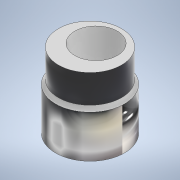
# Autodesk Inventor part: interior
Saved by Autodesk Inventor 2021 (Build 250183000, 183)
## iProperties
Created: 2022-10-29
Part Number: interior
Material: Genérico
Document SubType Name: Modeling
Designer: sergi
Density: 1 g/cm^3
Appearance: Valor por defecto
Author: sergi
Autodesk Inventor part; units mm, degrees
ref_plane "YZ Plane" through (0, 0, 0) normal (1, 0, 0) x (0, 1, 0)
ref_plane "XZ Plane" through (0, 0, 0) normal (0, 1, 0) x (-1, 0, 0)
ref_plane "XY Plane" through (0, 0, 0) normal (0, 0, 1) x (1, 0, 0)
sketch "Boceto1" plane through (0, 0, 0) normal (0, 1, 0) x (-1, 0, 0)
  circle A0 centre (0, 0) radius 4.05
  dimension "d0" = 8.1
  constraints: 1 centre point, 1 coincident
  measures "d0" diameter of A0
extrude "Extrusión1" add sketch "Boceto1" along normal blind 5
sketch "Boceto2" plane through (0, 5, 0) normal (0, 1, 0) x (1, 0, 0)
  circle A0 centre (0, 0) radius 3.715
  dimension "d3" = 7.43
  constraints: 1 centre point, 1 coincident
  measures "d3" diameter of A0
extrude "Extrusión2" add sketch "Boceto2" along normal blind 3.8
fillet "Empalme2" radius 0.5 1 edges at (-3.715, 5, 0)
sketch "Boceto14" plane through (0, 8.8, 0) normal (0, 1, 0) x (1, 0, 0)
  circle A0 centre (0, 0) radius 3.715 projected
  line L0 (0, 3.715) -> (0, 3.215)
  line L1 (0, 3.215) -> (0, 0.715)
  circle A1 centre (0, 0.715) radius 2.5
  dimension "d72" = 0.5
  dimension "d73" = 2.5
  constraints: 4 end point, 2 vertical, 2 vertical alignment, 1 coincident, 3 other
  measures "d72" distance of L0.start L0.end
  measures "d73" distance of L0.end L1.end
extrude "Extrusión7" cut sketch "Boceto14" against normal through all contours A1
equation "\"d23\" = 55deg"
equation "\"Boceto5_Pitch\" = 0.8"
equation "\"d45\" = 55deg"
equation "\"Boceto8_Pitch\" = 0.8"
